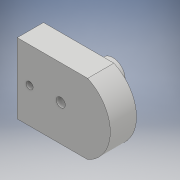
# Autodesk Inventor part: Część2
Saved by Autodesk Inventor 2017 SP1 (Build 210196100, 196)
## iProperties
Created: 2018-03-14
Part Number: Część2
Material: Ogólny
Document SubType Name: Modeling
Designer: student
Density: 1 g/cm^3
Appearance: Domyślna
Author: student
Autodesk Inventor part; units mm, degrees
ref_plane "YZ Plane" through (0, 0, 0) normal (1, 0, 0) x (0, 1, 0)
ref_plane "XZ Plane" through (0, 0, 0) normal (0, 1, 0) x (-1, 0, 0)
ref_plane "XY Plane" through (0, 0, 0) normal (0, 0, 1) x (1, 0, 0)
sketch "Szkic1" plane through (0, 0, 0) normal (0, 1, 0) x (-1, 0, 0)
  line L0 (8.460922, -2.595157) -> (8.460922, -202.595157)
  line L1 (8.460922, -202.595157) -> (-191.539078, -202.595157)
  line L2 (8.460922, -2.595157) -> (-191.539078, -2.595157)
  line L3 (8.460922, -2.595157) -> (208.460922, -2.595157) construction
  arc A0 (-191.539078, -2.595157) -> (-191.539078, -202.595157) centre (-145.713321, -102.595157) ccw
  line L4 (8.460922, -102.595157) -> (43.460922, -102.595157) construction
  circle A1 centre (-26.539078, -102.595157) radius 10
  point P0 (0, 0)
  dimension "d0" = 200
  dimension "d1" = 200
  dimension "d2" = 90
  dimension "d4" = 200
  dimension "d5" = 180
  dimension "d6" = 110
  dimension "d10" = 20
  constraints: 10 end point, 3 horizontal, 2 centre point, 2 point on circle, 1 collinear, 1 midpoint, 1 perpendicular, 1 vertical
  measures "d0" distance of L0.start L0.end
  measures "d1" distance of L0.end L1.end
  measures "d2" angle of L0 L1
  measures "d4" distance of L0.start L2.end
  measures "d5" angle of L2 L3
  measures "d6" radius of A0
  measures "d10" diameter of A1
extrude "Wyciągnięcie proste1" add sketch "Szkic1" along normal blind 74.5
sketch "Szkic2" plane through (0, 74.5, 0) normal (0, 1, 0) x (1, 0, 0)
  circle A0 centre (107.96185, 52.890403) radius 34.51232
  circle A1 centre (113.959733, 99.782925) radius 48.14156
  point P0 (0, 0)
  constraints: 2 centre point
sketch "Szkic2 outline for Wyciągnięcie proste2" plane through (0, 74.5, 0) normal (0, 1, 0) x (1, 0, 0)
  circle A0 centre (113.959733, 99.782925) radius 48.14156
extrude "Wyciągnięcie proste2" add sketch "Szkic2 outline for Wyciągnięcie proste2" along normal blind 74.5 draft -10
hole "Otwór1" at (114.99325, 149, -100.1379) direction (0, -1, 0) diameter 25.75 end through all
